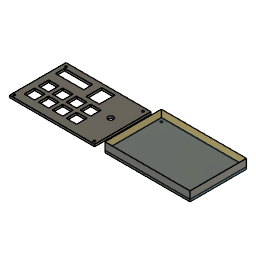
hackpad2 (Autodesk Fusion 360 design; units mm, degrees)
part number: 2026-03-07-22-10-30-789
Autodesk Fusion 360 part; units mm, degrees
note: some values were not read from the file. Set by a fixed rule: the direction of a hole.
sketch "Sketch1" plane through (0, 0, 0) normal (0, 0, 1) x (1, 0, 0)
  line L0 (-50, 50) -> (66, 50)
  line L1 (66, 50) -> (66, -27)
  line L2 (66, -27) -> (-50, -27)
  line L3 (-50, -27) -> (-50, 50)
  circle A0 centre (-45, 45) radius 1.45
  point P0 (-45, 45)
  dimension "d1" = 116
  dimension "d2" = 77
  dimension "d3" = 2.9
  constraint horizontal L0
  constraint vertical L1
  constraint horizontal L2
  constraint vertical L3
  measures "d1" distance of L0.start L0.end
  measures "d2" distance of L0.start L2.end
  measures "d3" diameter of A0
  measures "d4" diameter of A0
sketch "Sketch2" plane through (0, 0, 0) normal (0, 0, 1) x (1, 0, 0)
  circle A0 centre (60, 45) radius 1.45
  circle A1 centre (-45.3549, -21.776) radius 1.45
  circle A2 centre (60.8582, -21.4366) radius 1.45
  dimension "d4" = 2.9
  dimension "d5" = 2.9
  dimension "d6" = 2.9
  measures "d4" diameter of A0
  measures "d5" diameter of A1
  measures "d6" diameter of A2
sketch "Sketch3" plane through (0, 0, 0) normal (0, 0, 1) x (1, 0, 0)
extrude "Extrude1" add sketch "Sketch1" along normal blind 3 makes body 1
hole "Hole1" at (60, 45, 0) direction (0, 0, 1) diameter 2.9 depth 3 tip angle 118 bodies 1
hole "Hole2" at (61.9937, -23.3917, 3) direction (0, 0, -1) diameter 2.9 depth 3 tip angle 118 bodies 1
hole "Hole3" at (-47.1164, -23.4493, 3) direction (0, 0, -1) diameter 2.9 depth 3 tip angle 118 bodies 1
sketch "Sketch4" plane through (0, 0, 3) normal (0, 0, 1) x (-1, 0, 0)
  circle A0 centre (47.1164, 23.4493) radius 1.45
  circle A1 centre (-61.9937, 23.3917) radius 1.45
  circle A2 centre (-60, -45) radius 1.45
  circle A3 centre (45, -45) radius 1.45
  line L0 (50, 27) -> (-66, 27)
  line L1 (-66, 27) -> (-66, -50)
  line L2 (-66, -50) -> (50, -50)
  line L3 (50, -50) -> (50, 27)
sketch "Sketch5" plane through (66, 0, 0) normal (1, 0, 0) x (0, 1, 0)
  line L0 (-27, 0) -> (50, 0)
  line L1 (50, 0) -> (50, 3)
  line L2 (50, 3) -> (-27, 3)
  line L3 (-27, 3) -> (-27, 0)
surface "Extrude2" add extruded along (0, 0, 1) between 0 and 10 path "Sketch4" along L0 L1 L2 L3 separate body makes body 2
sketch "Sketch6" plane through (0, 0, 3) normal (0, 0, 1) x (-1, 0, 0)
  circle A0 centre (47.1164, 23.4493) radius 1.45
  circle A1 centre (-61.9937, 23.3917) radius 1.45
  circle A2 centre (-60, -45) radius 1.45
  circle A3 centre (45, -45) radius 1.45
  line L0 (50, 27) -> (-66, 27)
  line L1 (-66, 27) -> (-66, -50)
  line L2 (-66, -50) -> (50, -50)
  line L3 (50, -50) -> (50, 27)
copy_body "CopyPasteBodies1" bodies 1 makes body 3
move_body "Move1" bodies 3 to x (1, 0, 0) y (0, 1, 0) z (0, 0, 1) at (-290, 0, 0)
sketch "Sketch7" plane through (0, 0, 3) normal (0, 0, 1) x (-1, 0, 0)
  circle A0 centre (337.1164, 23.4493) radius 1.45
  circle A1 centre (228.0063, 23.3917) radius 1.45
  circle A2 centre (230, -45) radius 1.45
  circle A3 centre (335, -45) radius 1.45
  line L0 (340, 27) -> (224, 27)
  line L1 (224, 27) -> (224, -50)
  line L2 (224, -50) -> (340, -50)
  line L3 (340, -50) -> (340, 27)
  line L4 (336.45, -45) -> (229.37, -45)
  line L5 (229.37, -45) -> (229.37, 22.4)
  line L6 (229.37, 22.4) -> (336.45, 22.4)
  line L7 (336.45, 22.4) -> (336.45, -45)
  line L8 (260.525, 15.475) -> (273.525, 15.475)
  line L9 (260.525, 1.475) -> (273.525, 1.475)
  line L10 (260.025, 14.975) -> (260.025, 1.975)
  line L11 (274.025, 14.975) -> (274.025, 1.975)
  arc A4 (260.525, 15.475) -> (260.025, 14.975) centre (260.525, 14.975) ccw
  arc A5 (274.025, 14.975) -> (273.525, 15.475) centre (273.525, 14.975) ccw
  arc A6 (260.025, 1.975) -> (260.525, 1.475) centre (260.525, 1.975) ccw
  arc A7 (273.525, 1.475) -> (274.025, 1.975) centre (273.525, 1.975) ccw
  line L12 (279.575, 15.475) -> (292.575, 15.475)
  line L13 (279.575, 1.475) -> (292.575, 1.475)
  line L14 (279.075, 14.975) -> (279.075, 1.975)
  line L15 (293.075, 14.975) -> (293.075, 1.975)
  arc A8 (279.575, 15.475) -> (279.075, 14.975) centre (279.575, 14.975) ccw
  arc A9 (293.075, 14.975) -> (292.575, 15.475) centre (292.575, 14.975) ccw
  arc A10 (279.075, 1.975) -> (279.575, 1.475) centre (279.575, 1.975) ccw
  arc A11 (292.575, 1.475) -> (293.075, 1.975) centre (292.575, 1.975) ccw
  line L16 (298.625, 15.475) -> (311.625, 15.475)
  line L17 (298.625, 1.475) -> (311.625, 1.475)
  line L18 (298.125, 14.975) -> (298.125, 1.975)
  line L19 (312.125, 14.975) -> (312.125, 1.975)
  arc A12 (298.625, 15.475) -> (298.125, 14.975) centre (298.625, 14.975) ccw
  arc A13 (312.125, 14.975) -> (311.625, 15.475) centre (311.625, 14.975) ccw
  arc A14 (298.125, 1.975) -> (298.625, 1.475) centre (298.625, 1.975) ccw
  arc A15 (311.625, 1.475) -> (312.125, 1.975) centre (311.625, 1.975) ccw
  line L20 (317.675, 15.475) -> (330.675, 15.475)
  line L21 (317.675, 1.475) -> (330.675, 1.475)
  line L22 (317.175, 14.975) -> (317.175, 1.975)
  line L23 (331.175, 14.975) -> (331.175, 1.975)
  arc A16 (317.675, 15.475) -> (317.175, 14.975) centre (317.675, 14.975) ccw
  arc A17 (331.175, 14.975) -> (330.675, 15.475) centre (330.675, 14.975) ccw
  arc A18 (317.175, 1.975) -> (317.675, 1.475) centre (317.675, 1.975) ccw
  arc A19 (330.675, 1.475) -> (331.175, 1.975) centre (330.675, 1.975) ccw
  line L24 (260.525, -3.575) -> (273.525, -3.575)
  line L25 (260.525, -17.575) -> (273.525, -17.575)
  line L26 (260.025, -4.075) -> (260.025, -17.075)
  line L27 (274.025, -4.075) -> (274.025, -17.075)
  arc A20 (260.525, -3.575) -> (260.025, -4.075) centre (260.525, -4.075) ccw
  arc A21 (274.025, -4.075) -> (273.525, -3.575) centre (273.525, -4.075) ccw
  arc A22 (260.025, -17.075) -> (260.525, -17.575) centre (260.525, -17.075) ccw
  arc A23 (273.525, -17.575) -> (274.025, -17.075) centre (273.525, -17.075) ccw
  line L28 (279.575, -3.575) -> (292.575, -3.575)
  line L29 (279.575, -17.575) -> (292.575, -17.575)
  line L30 (279.075, -4.075) -> (279.075, -17.075)
  line L31 (293.075, -4.075) -> (293.075, -17.075)
  arc A24 (279.575, -3.575) -> (279.075, -4.075) centre (279.575, -4.075) ccw
  arc A25 (293.075, -4.075) -> (292.575, -3.575) centre (292.575, -4.075) ccw
  arc A26 (279.075, -17.075) -> (279.575, -17.575) centre (279.575, -17.075) ccw
  arc A27 (292.575, -17.575) -> (293.075, -17.075) centre (292.575, -17.075) ccw
  line L32 (298.625, -3.575) -> (311.625, -3.575)
  line L33 (298.625, -17.575) -> (311.625, -17.575)
  line L34 (298.125, -4.075) -> (298.125, -17.075)
  line L35 (312.125, -4.075) -> (312.125, -17.075)
  arc A28 (298.625, -3.575) -> (298.125, -4.075) centre (298.625, -4.075) ccw
  arc A29 (312.125, -4.075) -> (311.625, -3.575) centre (311.625, -4.075) ccw
  arc A30 (298.125, -17.075) -> (298.625, -17.575) centre (298.625, -17.075) ccw
  arc A31 (311.625, -17.575) -> (312.125, -17.075) centre (311.625, -17.075) ccw
  line L36 (317.675, -3.575) -> (330.675, -3.575)
  line L37 (317.675, -17.575) -> (330.675, -17.575)
  line L38 (317.175, -4.075) -> (317.175, -17.075)
  line L39 (331.175, -4.075) -> (331.175, -17.075)
  arc A32 (317.675, -3.575) -> (317.175, -4.075) centre (317.675, -4.075) ccw
  arc A33 (331.175, -4.075) -> (330.675, -3.575) centre (330.675, -4.075) ccw
  arc A34 (317.175, -17.075) -> (317.675, -17.575) centre (317.675, -17.075) ccw
  arc A35 (330.675, -17.575) -> (331.175, -17.075) centre (330.675, -17.075) ccw
  line L40 (257.5, -20.1) -> (333.7, -20.1)
  line L41 (257.5, 18) -> (333.7, 18)
  line L42 (257.5, -20.1) -> (257.5, 18)
  line L43 (333.7, -20.1) -> (333.7, 18)
  circle A36 centre (244, -15) radius 3.6
  line L44 (334, -42) -> (296, -42)
  line L45 (296, -42) -> (296, -30)
  line L46 (296, -30) -> (334, -30)
  line L47 (334, -30) -> (334, -42)
  line L48 (286.075, -44.6768) -> (268.275, -44.6768)
  line L49 (268.275, -44.6768) -> (268.275, -23.6768)
  line L50 (268.275, -23.6768) -> (286.075, -23.6768)
  line L51 (286.075, -23.6768) -> (286.075, -44.6768)
  dimension "d24" = 107.08
  dimension "d25" = 67.4
  dimension "d26" = 7.2
  dimension "d27" = 38
  dimension "d28" = 12
  dimension "d29" = 17.8
  dimension "d30" = 21
  constraint horizontal L4
  constraint vertical L5
  constraint horizontal L6
  constraint vertical L7
  constraint coincident A3 L4.start
  constraint horizontal L44
  constraint vertical L45
  constraint horizontal L46
  constraint vertical L47
  constraint horizontal L48
  constraint vertical L49
  constraint horizontal L50
  constraint vertical L51
  measures "d24" distance of L4.start L4.end
  measures "d25" distance of L4.start L6.end
  measures "d26" diameter of A36
  measures "d27" distance of L44.start L44.end
  measures "d28" distance of L44.start L46.end
  measures "d29" distance of L48.start L48.end
  measures "d30" distance of L48.start L50.end
form "Form1" [no effect]
extrude "Extrude3" cut sketch "Sketch7" against normal blind 3 contours L8 L9 L10 L11 A4 A5 A6 A7 | L12 L13 L14 L15 A8 A9 A10 A11 | L16 L17 L18 L19 A12 A13 A14 A15 | L20 L21 L22 L23 A16 A17 A18 A19 | L24 L25 L26 L27 A20 A21 A22 A23 | L28 L29 L30 L31 A24 A25 A26 A27 | L32 L33 L34 L35 A28 A29 A30 A31 | L36 L37 L38 L39 A32 A33 A34 A35 | A36 | L44 L45 L46 L47 | L48 L49 L50 L51 bodies 3
sketch "Sketch8" plane through (0, 0, 3) normal (0, 0, 1) x (-1, 0, 0)
move_body "Move2" bodies 3 to x (1, 0, 0) y (0, 1, 0) z (0, 0, 1) at (160, 0, 0)
